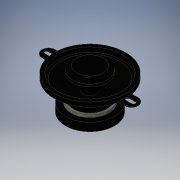
# Autodesk Inventor part: Speaker_Massive_MX3
Saved by Autodesk Inventor 2016 (Build 200138000, 138)
## iProperties
Created: 2019-09-19
Part Number: Speaker_Massive_MX3
Material: Generic
Document SubType Name: Modeling
Designer: jimmy
Density: 1 g/cm^3
Appearance: Default
Author: jimmy
Autodesk Inventor part; units mm, degrees
ref_plane "YZ Plane" through (0, 0, 0) normal (1, 0, 0) x (0, 1, 0)
ref_plane "XZ Plane" through (0, 0, 0) normal (0, 1, 0) x (-1, 0, 0)
ref_plane "XY Plane" through (0, 0, 0) normal (0, 0, 1) x (1, 0, 0)
sketch "Sketch1" plane through (0, 0, 0) normal (0, 0, 1) x (1, 0, 0)
  circle A0 centre (0, 0) radius 43.5
  circle A1 centre (0, 0) radius 39
  dimension "d0" = 87
  dimension "d1" = 78
  constraints: 2 centre point, 2 coincident
  measures "d0" diameter of A0
  measures "d1" diameter of A1
extrude "Extrusion1" add sketch "Sketch1" along normal blind 5.5
sketch "Sketch2" plane through (0, 0, 0) normal (0, 1, 0) x (-1, 0, 0)
  line L0 (43.5, 5.5) -> (-43.5, 5.5) projected
  line L1 (-43.5, 0) -> (43.5, 0) projected
  line L2 (43.5, 0) -> (43.5, 5.5) projected
  line L3 (-43.5, 0) -> (-43.5, 5.5) projected
  line L4 (0, -1.1) -> (0, 6.6) construction
  line L5 (0, 0) -> (0, -38.5) construction
  line L6 (0, -38.5) -> (-30, -38.5)
  line L7 (-30, -38.5) -> (-30, -22.5)
  line L8 (-30, -22.5) -> (0, -22.5)
  line L9 (0, -22.5) -> (0, -38.5)
  line L10 (-30, -22.5) -> (-23, -22.5)
  line L11 (-23, -22.5) -> (-23, -25.5)
  line L12 (-23, -25.5) -> (-30, -25.5)
  line L13 (-30, -25.5) -> (-30, -22.5)
  line L14 (-30, -38.5) -> (-23, -38.5)
  line L15 (-23, -38.5) -> (-23, -35.5)
  line L16 (-23, -35.5) -> (-30, -35.5)
  line L17 (-30, -35.5) -> (-30, -38.5)
  line L18 (-39, 0) -> (-39, 5.5) projected
  line L19 (-39, 0) -> (-36, 0)
  line L20 (-43.5, 0) -> (43.5, 0) projected
  line L21 (-36, 0) -> (0, -16.7363)
  line L22 (0, -16.7363) -> (0, -22.5)
  line L23 (-39, 0) -> (-20.2226, -22.5)
  dimension "d4" = 38.5
  dimension "d5" = 30
  dimension "d6" = 16
  dimension "d7" = 7
  dimension "d8" = 3
  dimension "d9" = 7
  dimension "d10" = 3
  dimension "d11" = 3
  constraints: 34 end point, 6 parallel, 4 point on line, 3 horizontal, 3 perpendicular, 1 collinear
  measures "d4" distance of L5.start L5.end
  measures "d5" distance of L7.end L8.end
  measures "d6" distance of L6.end L7.end
  measures "d7" distance of L11.end L12.end
  measures "d8" distance of L10.end L11.end
  measures "d9" distance of L16.end L15.end
  measures "d10" distance of L15.end L14.end
  measures "d11" distance of L18.start L19.end
revolve "Revolution1" add sketch "Sketch2" angle 360 about axis through (0, 0, 0) along (0, 0, -1) contours L1 L21 L22 L8 L23 | L8 L9 L6 L15 L16 L7 L12 L11
sketch "Sketch3" plane through (0, 0, 0) normal (0, 1, 0) x (-1, 0, 0)
  line L0 (0, -47.3) -> (0, 14.3) construction
  line L1 (30, -35.5) -> (-30, -35.5) projected
  line L2 (-30, -25.5) -> (30, -25.5) projected
  line L3 (-30, -25.5) -> (30, -25.5) projected
  line L4 (0, -25.5) -> (-8, -25.5)
  line L5 (-8, -25.5) -> (-8, 5.5)
  line L6 (-8, 5.5) -> (0, 5.5)
  line L7 (0, 5.5) -> (0, -25.5)
  line L8 (0, 5.5) -> (-21, 5.5)
  line L9 (-21, 5.5) -> (-21, 13.5)
  line L10 (-21, 13.5) -> (0, 13.5)
  line L11 (0, 13.5) -> (0, 5.5)
  point P0 (0, 0)
  dimension "d13" = 8
  dimension "d14" = 31
  dimension "d15" = 21
  dimension "d16" = 8
  constraints: 16 end point, 4 parallel, 2 horizontal, 2 perpendicular, 1 midpoint
  measures "d13" distance of L5.end L6.end
  measures "d14" distance of L4.end L5.end
  measures "d15" distance of L9.end L10.end
  measures "d16" distance of L8.end L9.end
revolve "Revolution2" add sketch "Sketch3" angle 360 about axis through (0, 0, -10) along (0, 0, 1)
sketch "Sketch4" plane through (0, 0, 0) normal (0, 0, -1) x (-1, 0, 0)
  circle A0 centre (0, 0) radius 43.5 projected
  line L0 (60.9, 0) -> (-60.9, 0) construction
  line L1 (0, -60.9) -> (0, 60.9) construction
  line L2 (52, 0) -> (-52, 0)
  line L3 (46.2174, 0) -> (53.2174, 0) construction
  line L4 (46.2174, -2.435) -> (53.2174, -2.435)
  line L5 (53.2174, 2.435) -> (46.2174, 2.435)
  arc A1 (46.2174, 2.435) -> (46.2174, -2.435) centre (46.2174, 0) ccw
  arc A2 (53.2174, -2.435) -> (53.2174, 2.435) centre (53.2174, 0) ccw
  circle A3 centre (0, 0) radius 43.5 projected
  line L6 (42.758, -8) -> (50.6871, -8)
  line L7 (42.758, 8) -> (50.6871, 8)
  arc A4 (50.6871, -8) -> (50.6871, 8) centre (50.6871, 0) ccw
  point P0 (49.7174, 0)
  dimension "d18" = 104
  dimension "d19" = 3.5
  dimension "d20" = 4.87
  dimension "d21" = 8
  dimension "d22" = 8
  constraints: 14 end point, 10 point on circle, 6 tangent, 4 point on line, 3 centre point, 2 horizontal, 2 midpoint, 1 collinear, 1 parallel
  measures "d18" distance of L2.start L2.end
  measures "d19" distance of point (49.717, 0) L3.end
  measures "d20" diameter of A2
  measures "d21" distance between parallel lines of L6 L3
  measures "d22" distance between parallel lines of L3 L7
extrude "Extrusion2" add sketch "Sketch4" against normal blind 1 contours A0 L7 A4 L6
mirror "Mirror1" about plane through (0, 0, 0) normal (1, 0, 0) of "Extrusion2"
fillet "Fillet1" radius 5 1 edges at (-21, 0, 13.5)
body "Solid1"
